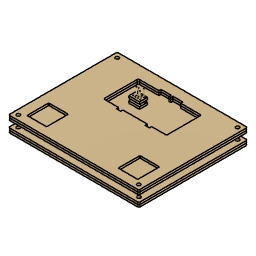
Solum Newton M3 4.3 - Fusion360 (Autodesk Fusion 360 design; units mm, degrees)
Autodesk Fusion 360 part; units mm, degrees
sketch "Skizze1" plane through (0, 0, 0) normal (0, 0, 1) x (1, 0, 0)
  line L0 (-29, 42) -> (-29, 12)
  line L1 (29, 12) -> (29, 42)
  line L2 (-10, 43) -> (-10, 45)
  line L3 (10, 43) -> (10, 45)
  line L4 (10, 45) -> (0.8, 45)
  line L5 (-10, 45) -> (-0.8, 45)
  line L6 (-0.8, 45) -> (-0.8, 43)
  line L7 (0.8, 45) -> (0.8, 43)
  line L8 (-15.25, 9) -> (-15.25, 11)
  line L9 (15.25, 11) -> (15.25, 9)
  line L10 (-11.25, 9) -> (-11.25, 11)
  line L11 (11.25, 11) -> (11.25, 9)
  line L12 (15.25, 9) -> (11.25, 9)
  line L13 (-11.25, 9) -> (-15.25, 9)
  line L14 (15.25, 11) -> (28, 11)
  line L15 (-28, 11) -> (-15.25, 11)
  line L16 (-11.25, 11) -> (11.25, 11)
  arc A0 (-28, 43) -> (-29, 42) centre (-28, 42) ccw
  arc A1 (29, 42) -> (28, 43) centre (28, 42) ccw
  arc A2 (28, 11) -> (29, 12) centre (28, 12) ccw
  arc A3 (-29, 12) -> (-28, 11) centre (-28, 12) ccw
  line L17 (-50.5, -17.5) -> (-33.5, -17.5)
  line L18 (-33, -18) -> (-33, -37)
  line L19 (-33.5, -37.5) -> (-50.5, -37.5)
  line L20 (-51, -37) -> (-51, -18)
  line L21 (51.5, 46) -> (-51.5, 46) construction
  line L22 (-51.5, 46) -> (-51.5, -37) construction
  line L23 (-51.5, -37) -> (51.5, -37) construction
  line L24 (51.5, -37) -> (51.5, 46) construction
  line L25 (51.5, 46) -> (-51.5, -37) construction
  line L26 (-51.5, 46) -> (51.5, -37) construction
  line L27 (50.5, -37.5) -> (33.5, -37.5)
  line L28 (33, -37) -> (33, -18)
  line L29 (33.5, -17.5) -> (50.5, -17.5)
  line L30 (51, -18) -> (51, -37)
  line L31 (-14.05, 36.45) -> (-14.05, 29.15)
  circle A4 centre (-15.75, 35) radius 0.75
  circle A5 centre (-19.95, 35) radius 0.75
  circle A6 centre (-19.95, 31.4) radius 0.75
  circle A7 centre (-16.75, 33.2) radius 0.75
  circle A8 centre (-15.75, 31.4) radius 0.75
  line L32 (-23.85, 36.45) -> (-14.05, 36.45)
  circle A9 centre (-17.85, 31.4) radius 0.75
  circle A10 centre (-17.85, 35) radius 0.75
  line L33 (-23.85, 29.15) -> (-14.05, 36.45) construction
  circle A11 centre (-20.95, 33.2) radius 0.75
  circle A12 centre (-18.85, 33.2) radius 0.75
  circle A13 centre (-22.05, 35) radius 0.75
  circle A14 centre (-22.05, 31.4) radius 0.75
  line L34 (-14.05, 29.15) -> (-23.85, 36.45) construction
  line L35 (-23.85, 29.15) -> (-23.85, 36.45)
  line L36 (-14.05, 29.15) -> (-23.85, 29.15)
  line L37 (59, -45.5) -> (-59, -45.5)
  line L38 (-60, -44.5) -> (-60, 53.5)
  line L39 (-59, 54.5) -> (59, 54.5)
  line L40 (60, 53.5) -> (60, -44.5)
  line L41 (60, -45.5) -> (-60, 54.5) construction
  line L42 (-60, -45.5) -> (60, 54.5) construction
  circle A15 centre (-55.5, 50) radius 1.6
  circle A16 centre (55.5, 50) radius 1.6
  circle A17 centre (-55.5, -41) radius 1.6
  circle A18 centre (55.5, -41) radius 1.6
  line L43 (-10, 43) -> (-28, 43)
  line L44 (28, 43) -> (10, 43)
  line L45 (0.8, 43) -> (-0.8, 43)
  arc A19 (-59, 54.5) -> (-60, 53.5) centre (-59, 53.5) ccw
  arc A20 (60, 53.5) -> (59, 54.5) centre (59, 53.5) ccw
  arc A21 (-60, -44.5) -> (-59, -45.5) centre (-59, -44.5) ccw
  arc A22 (59, -45.5) -> (60, -44.5) centre (59, -44.5) ccw
  arc A23 (-50.5, -17.5) -> (-51, -18) centre (-50.5, -18) ccw
  arc A24 (-33, -18) -> (-33.5, -17.5) centre (-33.5, -18) ccw
  arc A25 (-51, -37) -> (-50.5, -37.5) centre (-50.5, -37) ccw
  arc A26 (-33.5, -37.5) -> (-33, -37) centre (-33.5, -37) ccw
  arc A27 (33.5, -17.5) -> (33, -18) centre (33.5, -18) ccw
  arc A28 (33, -37) -> (33.5, -37.5) centre (33.5, -37) ccw
  arc A29 (51, -18) -> (50.5, -17.5) centre (50.5, -18) ccw
  arc A30 (50.5, -37.5) -> (51, -37) centre (50.5, -37) ccw
  circle A31 centre (-22.05, 35) radius 0.45
  circle A32 centre (-19.95, 35) radius 0.45
  circle A33 centre (-17.85, 35) radius 0.45
  circle A34 centre (-15.75, 35) radius 0.45
  circle A35 centre (-20.95, 33.2) radius 0.45
  circle A36 centre (-18.85, 33.2) radius 0.45
  circle A37 centre (-16.75, 33.2) radius 0.45
  circle A38 centre (-22.05, 31.4) radius 0.45
  circle A39 centre (-19.95, 31.4) radius 0.45
  circle A40 centre (-17.85, 31.4) radius 0.45
  circle A41 centre (-15.75, 31.4) radius 0.45
  line L46 (-14.05, 36.45) -> (-14.05, 43)
  line L47 (-23.85, 36.45) -> (-23.85, 43)
  point P0 (0, 27)
  point P1 (0, 11)
  point P2 (-51, -17.5)
  point P3 (-33, -17.5)
  point P4 (-51, -37.5)
  point P5 (0, 4.5)
  point P6 (51, -17.5)
  point P7 (33, -37.5)
  point P8 (33, -17.5)
  point P9 (-18.95, 32.8)
  point P10 (-18.95, 32.8)
  point P11 (0, 4.5)
  dimension "d6" = 2
  dimension "d7" = 9.2
  dimension "d8" = 9.2
  dimension "d22" = 1
  dimension "d23" = 1
  dimension "d24" = 1
  dimension "d25" = 1
  dimension "d43" = 18
  dimension "d44" = 20
  dimension "d45" = 103
  dimension "d46" = 83
  dimension "d47" = 18
  dimension "d48" = 20
  dimension "d54" = 9.8
  dimension "d55" = 7.3
  dimension "d56" = 1.5
  dimension "d57" = 120
  dimension "d58" = 100
  dimension "d59" = 3.2
  dimension "d60" = 3.2
  dimension "d61" = 3.2
  dimension "d62" = 3.2
  dimension "d69" = 1
  dimension "d70" = 1
  dimension "d71" = 1
  dimension "d72" = 1
  dimension "d73" = 0.5
  dimension "d74" = 0.5
  dimension "d75" = 0.5
  dimension "d76" = 0.5
  dimension "d77" = 0.5
  dimension "d78" = 0.5
  dimension "d79" = 0.5
  dimension "d80" = 0.5
  dimension "d89" = 0.9
  constraint horizontal L44
  constraint perpendicular L0 L44
  constraint parallel L15 L44
  constraint parallel L0 L1
  constraint coincident L2.start L44
  constraint perpendicular L2 L44
  constraint perpendicular L3 L44
  constraint perpendicular L3 L4
  constraint perpendicular L2 L5
  constraint perpendicular L5 L6
  constraint perpendicular L4 L7
  constraint horizontal L12
  constraint perpendicular L8 L12
  constraint coincident L9.start L15
  constraint collinear L12 L13
  constraint collinear L14 L15
  constraint coincident P1 L15
  constraint collinear L15 L16
  constraint tangent A0 L44
  constraint tangent L0 A0
  constraint tangent A1 L44
  constraint tangent L1 A1
  constraint tangent L14 A2
  constraint tangent L1 A2
  constraint tangent L0 A3
  constraint tangent L15 A3
  constraint horizontal L17
  constraint vertical L18
  constraint horizontal L19
  constraint vertical L20
  constraint horizontal L21
  constraint perpendicular L21 L22
  constraint parallel L21 L23
  constraint parallel L22 L24
  constraint coincident L25 P11
  constraint coincident L26 P11
  constraint horizontal L29
  constraint vertical L30
  constraint horizontal L27
  constraint vertical L28
  constraint horizontal L36
  constraint perpendicular L35 L36
  constraint parallel L32 L36
  constraint parallel L31 L35
  constraint coincident P10 L34
  constraint coincident P10 L33
  constraint coincident P10 P9
  constraint equal A5 A13
  constraint equal A10 A13
  constraint equal A4 A13
  constraint equal A12 A13
  constraint equal A7 A13
  constraint equal A13 A14
  constraint equal A9 A13
  constraint equal A8 A13
  constraint horizontal L37
  constraint perpendicular L37 L38
  constraint parallel L37 L39
  constraint parallel L38 L40
  constraint coincident L41 P11
  constraint coincident L42 P11
  constraint coincident P11 P5
  constraint collinear L43 L44
  constraint collinear L44 L45
  constraint coincident L41.end L39
  constraint coincident L41.end L38
  constraint tangent L39 A19
  constraint tangent L38 A19
  constraint coincident L42.end L39
  constraint coincident L42.end L40
  constraint tangent L39 A20
  constraint tangent L40 A20
  constraint coincident L42.start L38
  constraint coincident L42.start L37
  constraint tangent L38 A21
  constraint tangent L37 A21
  constraint coincident L41.start L37
  constraint coincident L41.start L40
  constraint tangent L37 A22
  constraint tangent L40 A22
  constraint coincident P2 L17
  constraint coincident P2 L20
  constraint tangent L17 A23
  constraint tangent L20 A23
  constraint coincident P3 L17
  constraint coincident P3 L18
  constraint tangent L17 A24
  constraint tangent L18 A24
  constraint coincident P4 L20
  constraint coincident P4 L19
  constraint tangent L20 A25
  constraint tangent L19 A25
  constraint tangent L19 A26
  constraint tangent L18 A26
  constraint coincident P8 L28
  constraint coincident P8 L29
  constraint tangent L28 A27
  constraint tangent L29 A27
  constraint coincident P7 L28
  constraint coincident P7 L27
  constraint tangent L28 A28
  constraint tangent L27 A28
  constraint coincident P6 L29
  constraint coincident P6 L30
  constraint tangent L29 A29
  constraint tangent L30 A29
  constraint tangent L27 A30
  constraint tangent L30 A30
  constraint concentric A13 A31
  constraint concentric A5 A32
  constraint concentric A10 A33
  constraint concentric A4 A34
  constraint concentric A11 A35
  constraint concentric A12 A36
  constraint concentric A7 A37
  constraint concentric A14 A38
  constraint concentric A6 A39
  constraint concentric A9 A40
  constraint concentric A8 A41
  constraint equal A31 A32
  constraint equal A31 A33
  constraint equal A31 A34
  constraint equal A31 A35
  constraint equal A31 A36
  constraint equal A31 A37
  constraint equal A31 A38
  constraint equal A31 A39
  constraint equal A31 A40
  constraint equal A31 A41
  constraint coincident L43 L46.end
  constraint perpendicular L43 L46
  constraint coincident L43 L47.end
  constraint perpendicular L43 L47
  measures "d6" distance of L2.start L2.end
  measures "d7" distance of L3.end L4.end
  measures "d8" distance of L2.end L5.end
  measures "d22" radius of A0
  measures "d23" radius of A1
  measures "d24" radius of A2
  measures "d25" radius of A3
  measures "d43" distance of P2 P3
  measures "d44" distance of P2 P4
  measures "d45" distance of L22.end L23.end
  measures "d46" distance of L21.end L22.end
  measures "d47" distance of P6 P8
  measures "d48" distance of P7 P8
  measures "d54" distance of L31.start L32.start
  measures "d55" distance of L33.start L32.start
  measures "d56" diameter of A13
  measures "d57" distance of L41.end L42.end
  measures "d58" distance of L42.start L41.end
  measures "d59" diameter of A15
  measures "d60" diameter of A16
  measures "d61" diameter of A17
  measures "d62" diameter of A18
  measures "d69" radius of A19
  measures "d70" radius of A20
  measures "d71" radius of A21
  measures "d72" radius of A22
  measures "d73" radius of A23
  measures "d74" radius of A24
  measures "d75" radius of A25
  measures "d76" radius of A26
  measures "d77" radius of A27
  measures "d78" radius of A28
  measures "d79" radius of A29
  measures "d80" radius of A30
  measures "d89" diameter of A31
extrude "Extrusion20" add sketch "Skizze1" along normal blind 2 contours L0 L1 L2 L3 L4 L5 L6 L7 L8 L9 L10 L11 L12 L13 L14 L15 L16 A0 A1 A2 A3 L31 L35 L36 L43 L44 L45 L46 L47 | L32 L43 L46 L47 | L31 L32 L35 L36 | L17 L18 L19 L20 A23 A24 A25 A26 | L27 L28 L29 L30 A27 A28 A29 A30 | A4 | A5 | A6 | A7 | A8 | A9 | A10 | A11 | A12 | A13 | A14 | L37 L38 L39 L40 A19 A20 A21 A22 | A31 | A32 | A33 | A34 | A35 | A36 | A37 | A38 | A39 | A40 | A41 makes body 1
extrude "Extrusion21" add sketch "Skizze1" along normal blind 2 separate body contours L0 L1 L2 L3 L4 L5 L6 L7 L8 L9 L10 L11 L12 L13 L14 L15 L16 A0 A1 A2 A3 L31 L35 L36 L43 L44 L45 L46 L47 | L32 L43 L46 L47 | L31 L32 L35 L36 | L17 L18 L19 L20 A23 A24 A25 A26 | L27 L28 L29 L30 A27 A28 A29 A30 | A4 | A5 | A6 | A7 | A8 | A9 | A10 | A11 | A12 | A13 | A14 | L37 L38 L39 L40 A19 A20 A21 A22 makes body 2
move_body "Verschieben10" bodies 2 to x (1, 0, 0) y (0, 1, 0) z (0, 0, 1) at (0, 0, 2)
extrude "Extrusion25" add sketch "Skizze1" along normal blind 2 separate body contours L31 L32 L35 L36 | A4 | A5 | A6 | A7 | A8 | A9 | A10 | A11 | A12 | A13 | A14 makes body 3
move_body "Verschieben15" bodies 3 to x (1, 0, 0) y (0, 1, 0) z (0, 0, 1) at (0, 0, 4)
copy_body "Körper kopieren/einfügen4" bodies 3 makes body 4
move_body "Verschieben16" bodies 4 to x (1, 0, 0) y (0, 1, 0) z (0, 0, 1) at (0, 0, 4)
extrude "Extrusion26" add sketch "Skizze1" along normal blind 2 separate body contours L17 L18 L19 L20 A23 A24 A25 A26 | L27 L28 L29 L30 A27 A28 A29 A30 | L37 L38 L39 L40 A19 A20 A21 A22 makes body 5
move_body "Verschieben17" bodies 5 to x (1, 0, 0) y (0, 1, 0) z (0, 0, 1) at (0, 0, 10)
extrude "Extrusion27" add sketch "Skizze1" along normal blind 2 separate body contours L37 L38 L39 L40 A19 A20 A21 A22 makes body 6
move_body "Verschieben18" bodies 6 to x (1, 0, 0) y (0, 1, 0) z (0, 0, 1) at (0, 0, 12)
extrude "Extrusion28" add sketch "Skizze1" along normal blind 15 separate body contours A34 | A35 | A36 | A41 makes body 7 at (-16.1087, 31.6717, 10) makes body 8 at (-19.2978, 33.1552, 10) makes body 9 at (-15.3353, 35.1748, 10) makes body 10 at (-21.3978, 33.1552, 10)
move_body "Verschieben19" bodies 7 8 10 9 to x (1, 0, 0) y (0, 1, 0) z (0, 0, 1) at (0, 0, 2)
chamfer "Fase1" distance 0.3 angle 45 4 faces at (-15.5165, 34.9155, 17) (-18.8834, 33.3462, 17) (-15.8444, 31.6586, 17) (-20.9834, 33.3462, 17) on bodies 7 8 9 10
sketch "Skizze21" plane through (0, 0, 4) normal (0, 0, 1) x (-1, 0, 0)
  circle A0 centre (17.85, -31.4) radius 0.45
  circle A1 centre (18.85, -33.2) radius 0.45
  circle A2 centre (-55.5, -50) radius 1.6
  circle A3 centre (55.5, 41) radius 1.6
  circle A4 centre (22.05, -35) radius 0.45
  circle A5 centre (20.95, -33.2) radius 0.45
  circle A6 centre (19.95, -35) radius 0.45
  circle A7 centre (22.05, -31.4) radius 0.45
  circle A8 centre (15.75, -35) radius 0.45
  circle A9 centre (17.85, -35) radius 0.45
  circle A10 centre (15.75, -31.4) radius 0.45
  circle A11 centre (16.75, -33.2) radius 0.45
  circle A12 centre (55.5, -50) radius 1.6
  circle A13 centre (-55.5, 41) radius 1.6
  circle A14 centre (19.95, -31.4) radius 0.45
  arc A15 (60, 44.5) -> (59, 45.5) centre (59, 44.5) ccw
  line L0 (59, 45.5) -> (-59, 45.5)
  arc A16 (-59, 45.5) -> (-60, 44.5) centre (-59, 44.5) ccw
  line L1 (-60, 44.5) -> (-60, -53.5)
  arc A17 (-60, -53.5) -> (-59, -54.5) centre (-59, -53.5) ccw
  line L2 (-59, -54.5) -> (59, -54.5)
  arc A18 (59, -54.5) -> (60, -53.5) centre (59, -53.5) ccw
  line L3 (60, -53.5) -> (60, 44.5)
sketch "Skizze20" plane through (0, 0, 14) normal (0, 0, 1) x (-1, 0, 0)
  circle A0 centre (55.5, -50) radius 1.6
  line L0 (-28, -11) -> (-15.25, -11)
  line L1 (-15.25, -11) -> (-15.25, -9)
  line L2 (-15.25, -9) -> (-11.25, -9)
  line L3 (-11.25, -9) -> (-11.25, -11)
  line L4 (-11.25, -11) -> (11.25, -11)
  line L5 (11.25, -11) -> (11.25, -9)
  line L6 (11.25, -9) -> (15.25, -9)
  line L7 (15.25, -9) -> (15.25, -11)
  line L8 (15.25, -11) -> (28, -11)
  arc A1 (29, -12) -> (28, -11) centre (28, -12) ccw
  line L9 (29, -12) -> (29, -42)
  arc A2 (28, -43) -> (29, -42) centre (28, -42) ccw
  line L10 (28, -43) -> (10, -43)
  line L11 (10, -43) -> (10, -45)
  line L12 (10, -45) -> (0.8, -45)
  line L13 (0.8, -45) -> (0.8, -43)
  line L14 (0.8, -43) -> (-0.8, -43)
  line L15 (-0.8, -43) -> (-0.8, -45)
  line L16 (-0.8, -45) -> (-10, -45)
  line L17 (-10, -45) -> (-10, -43)
  line L18 (-10, -43) -> (-28, -43)
  arc A3 (-29, -42) -> (-28, -43) centre (-28, -42) ccw
  line L19 (-29, -42) -> (-29, -12)
  arc A4 (-28, -11) -> (-29, -12) centre (-28, -12) ccw
  circle A5 centre (-55.5, -50) radius 1.6
  arc A6 (51, 37) -> (50.5, 37.5) centre (50.5, 37) ccw
  line L20 (51, 37) -> (51, 18)
  arc A7 (50.5, 17.5) -> (51, 18) centre (50.5, 18) ccw
  line L21 (50.5, 17.5) -> (33.5, 17.5)
  arc A8 (33, 18) -> (33.5, 17.5) centre (33.5, 18) ccw
  line L22 (33, 18) -> (33, 37)
  arc A9 (33.5, 37.5) -> (33, 37) centre (33.5, 37) ccw
  line L23 (33.5, 37.5) -> (50.5, 37.5)
  circle A10 centre (55.5, 41) radius 1.6
  circle A11 centre (-55.5, 41) radius 1.6
  arc A12 (-33, 37) -> (-33.5, 37.5) centre (-33.5, 37) ccw
  line L24 (-33, 37) -> (-33, 18)
  arc A13 (-33.5, 17.5) -> (-33, 18) centre (-33.5, 18) ccw
  line L25 (-33.5, 17.5) -> (-50.5, 17.5)
  arc A14 (-51, 18) -> (-50.5, 17.5) centre (-50.5, 18) ccw
  line L26 (-51, 18) -> (-51, 37)
  arc A15 (-50.5, 37.5) -> (-51, 37) centre (-50.5, 37) ccw
  line L27 (-50.5, 37.5) -> (-33.5, 37.5)
  arc A16 (60, 44.5) -> (59, 45.5) centre (59, 44.5) ccw
  line L28 (59, 45.5) -> (-59, 45.5)
  arc A17 (-59, 45.5) -> (-60, 44.5) centre (-59, 44.5) ccw
  line L29 (-60, 44.5) -> (-60, -53.5)
  arc A18 (-60, -53.5) -> (-59, -54.5) centre (-59, -53.5) ccw
  line L30 (-59, -54.5) -> (59, -54.5)
  arc A19 (59, -54.5) -> (60, -53.5) centre (59, -53.5) ccw
  line L31 (60, -53.5) -> (60, 44.5)
sketch "Skizze19" plane through (0, 0, 12) normal (0, 0, 1) x (-1, 0, 0)
  line L0 (-28, -11) -> (-15.25, -11)
  line L1 (-15.25, -11) -> (-15.25, -9)
  line L2 (-15.25, -9) -> (-11.25, -9)
  line L3 (-11.25, -9) -> (-11.25, -11)
  line L4 (-11.25, -11) -> (11.25, -11)
  line L5 (11.25, -11) -> (11.25, -9)
  line L6 (11.25, -9) -> (15.25, -9)
  line L7 (15.25, -9) -> (15.25, -11)
  line L8 (15.25, -11) -> (28, -11)
  arc A0 (29, -12) -> (28, -11) centre (28, -12) ccw
  line L9 (29, -12) -> (29, -42)
  arc A1 (28, -43) -> (29, -42) centre (28, -42) ccw
  line L10 (28, -43) -> (10, -43)
  line L11 (10, -43) -> (10, -45)
  line L12 (10, -45) -> (0.8, -45)
  line L13 (0.8, -45) -> (0.8, -43)
  line L14 (0.8, -43) -> (-0.8, -43)
  line L15 (-0.8, -43) -> (-0.8, -45)
  line L16 (-0.8, -45) -> (-10, -45)
  line L17 (-10, -45) -> (-10, -43)
  line L18 (-10, -43) -> (-28, -43)
  arc A2 (-29, -42) -> (-28, -43) centre (-28, -42) ccw
  line L19 (-29, -42) -> (-29, -12)
  arc A3 (-28, -11) -> (-29, -12) centre (-28, -12) ccw
  circle A4 centre (-55.5, -50) radius 1.6
  circle A5 centre (55.5, -50) radius 1.6
  circle A6 centre (55.5, 41) radius 1.6
  circle A7 centre (-55.5, 41) radius 1.6
  arc A8 (60, 44.5) -> (59, 45.5) centre (59, 44.5) ccw
  line L20 (59, 45.5) -> (-59, 45.5)
  arc A9 (-59, 45.5) -> (-60, 44.5) centre (-59, 44.5) ccw
  line L21 (-60, 44.5) -> (-60, -53.5)
  arc A10 (-60, -53.5) -> (-59, -54.5) centre (-59, -53.5) ccw
  line L22 (-59, -54.5) -> (59, -54.5)
  arc A11 (59, -54.5) -> (60, -53.5) centre (59, -53.5) ccw
  line L23 (60, -53.5) -> (60, 44.5)
sketch "Skizze18" plane through (0, 0, 8) normal (0, 0, 1) x (-1, 0, 0)
  circle A0 centre (20.95, -35) radius 0.45
  circle A1 centre (18.85, -35) radius 0.45
  circle A2 centre (16.75, -31.4) radius 0.45
  circle A3 centre (23.05, -35) radius 0.45
  circle A4 centre (16.75, -35) radius 0.45
  circle A5 centre (18.85, -31.4) radius 0.45
  circle A6 centre (20.95, -31.4) radius 0.45
  circle A7 centre (19.85, -33.2) radius 0.45
  circle A8 centre (21.95, -33.2) radius 0.45
  circle A9 centre (17.75, -33.2) radius 0.45
  circle A10 centre (23.05, -31.4) radius 0.45
  line L0 (15.05, -29.15) -> (15.05, -36.45)
  line L1 (15.05, -36.45) -> (24.85, -36.45)
  line L2 (24.85, -36.45) -> (24.85, -29.15)
  line L3 (24.85, -29.15) -> (15.05, -29.15)
sketch "Skizze17" plane through (0, 0, 4) normal (0, 0, 1) x (-1, 0, 0)
  circle A0 centre (23.05, -31.4) radius 0.45
  circle A1 centre (23.05, -35) radius 0.45
  circle A2 centre (18.85, -35) radius 0.45
  circle A3 centre (-55.5, -50) radius 1.6
  circle A4 centre (55.5, 41) radius 1.6
  circle A5 centre (16.75, -31.4) radius 0.45
  circle A6 centre (16.75, -35) radius 0.45
  circle A7 centre (17.75, -33.2) radius 0.45
  circle A8 centre (20.95, -31.4) radius 0.45
  circle A9 centre (55.5, -50) radius 1.6
  circle A10 centre (19.85, -33.2) radius 0.45
  circle A11 centre (21.95, -33.2) radius 0.45
  circle A12 centre (18.85, -31.4) radius 0.45
  circle A13 centre (-55.5, 41) radius 1.6
  circle A14 centre (20.95, -35) radius 0.45
  arc A15 (60, 44.5) -> (59, 45.5) centre (59, 44.5) ccw
  line L0 (59, 45.5) -> (-59, 45.5)
  arc A16 (-59, 45.5) -> (-60, 44.5) centre (-59, 44.5) ccw
  line L1 (-60, 44.5) -> (-60, -53.5)
  arc A17 (-60, -53.5) -> (-59, -54.5) centre (-59, -53.5) ccw
  line L2 (-59, -54.5) -> (59, -54.5)
  arc A18 (59, -54.5) -> (60, -53.5) centre (59, -53.5) ccw
  line L3 (60, -53.5) -> (60, 44.5)
sketch "Skizze16" plane through (0, 0, 2) normal (0, 0, 1) x (-1, 0, 0)
  circle A0 centre (-55.5, -50) radius 1.6
  circle A1 centre (-55.5, 41) radius 1.6
  circle A2 centre (55.5, 41) radius 1.6
  circle A3 centre (55.5, -50) radius 1.6
  arc A4 (60, 44.5) -> (59, 45.5) centre (59, 44.5) ccw
  line L0 (59, 45.5) -> (-59, 45.5)
  arc A5 (-59, 45.5) -> (-60, 44.5) centre (-59, 44.5) ccw
  line L1 (-60, 44.5) -> (-60, -53.5)
  arc A6 (-60, -53.5) -> (-59, -54.5) centre (-59, -53.5) ccw
  line L2 (-59, -54.5) -> (59, -54.5)
  arc A7 (59, -54.5) -> (60, -53.5) centre (59, -53.5) ccw
  line L3 (60, -53.5) -> (60, 44.5)
extrude "Extrusion22" [suppressed]
move_body "Verschieben11" [suppressed]
extrude "Extrusion23" [suppressed]
move_body "Verschieben12" [suppressed]
extrude "Extrusion24" [suppressed]
move_body "Verschieben13" [suppressed]
copy_body "Körper kopieren/einfügen3" [suppressed]
move_body "Verschieben14" [suppressed]
extrude "Extrusion15" [suppressed]
copy_body "Körper kopieren/einfügen1" [suppressed]
move_body "Verschieben1" [suppressed]
extrude "Extrusion16" [suppressed]
move_body "Verschieben2" [suppressed]
move_body "Verschieben3" [suppressed]
extrude "Extrusion17" [suppressed]
move_body "Verschieben4" [suppressed]
copy_body "Körper kopieren/einfügen2" [suppressed]
move_body "Verschieben5" [suppressed]
extrude "Extrusion18" [suppressed]
move_body "Verschieben6" [suppressed]
move_body "Verschieben7" [suppressed]
extrude "Extrusion19" [suppressed]
delete_body "Körper entfernen1" bodies 11
move_body "Verschieben8" [suppressed]
move_body "Verschieben9" [suppressed]
extrude "Extrusion14" [suppressed]
extrude "Extrusion13" [suppressed]
sketch "Skizze15" plane through (0, 0, 2) normal (0, 0, 1) x (-1, 0, 0)
  circle A0 centre (-55.5, -50) radius 1.6
  circle A1 centre (-18.3, -33.2) radius 0.45
  circle A2 centre (-55.5, 41) radius 1.6
  circle A3 centre (-23.5, -31.4) radius 0.45
  circle A4 centre (55.5, -50) radius 1.6
  circle A5 centre (-17.2, -35) radius 0.45
  circle A6 centre (-21.4, -31.4) radius 0.45
  circle A7 centre (-19.3, -31.4) radius 0.45
  circle A8 centre (-21.4, -35) radius 0.45
  circle A9 centre (-22.5, -33.2) radius 0.45
  circle A10 centre (-17.2, -31.4) radius 0.45
  circle A11 centre (-19.3, -35) radius 0.45
  circle A12 centre (55.5, 41) radius 1.6
  circle A13 centre (-20.4, -33.2) radius 0.45
  circle A14 centre (-23.5, -35) radius 0.45
  arc A15 (60, 44.5) -> (59, 45.5) centre (59, 44.5) ccw
  line L0 (59, 45.5) -> (-59, 45.5)
  arc A16 (-59, 45.5) -> (-60, 44.5) centre (-59, 44.5) ccw
  line L1 (-60, 44.5) -> (-60, -53.5)
  arc A17 (-60, -53.5) -> (-59, -54.5) centre (-59, -53.5) ccw
  line L2 (-59, -54.5) -> (59, -54.5)
  arc A18 (59, -54.5) -> (60, -53.5) centre (59, -53.5) ccw
  line L3 (60, -53.5) -> (60, 44.5)
extrude "Extrusion12" [suppressed]
sketch "Skizze14" plane through (0, 0, 2) normal (0, 0, 1) x (-1, 0, 0)
  circle A0 centre (55.5, -50) radius 1.6
  circle A1 centre (-55.5, 41) radius 1.6
  circle A2 centre (55.5, 41) radius 1.6
  line L0 (-28, -11) -> (-15.25, -11)
  line L1 (-15.25, -11) -> (-15.25, -9)
  line L2 (-15.25, -9) -> (-11.25, -9)
  line L3 (-11.25, -9) -> (-11.25, -11)
  line L4 (-11.25, -11) -> (11.25, -11)
  line L5 (11.25, -11) -> (11.25, -9)
  line L6 (11.25, -9) -> (15.25, -9)
  line L7 (15.25, -9) -> (15.25, -11)
  line L8 (15.25, -11) -> (28, -11)
  arc A3 (29, -12) -> (28, -11) centre (28, -12) ccw
  line L9 (29, -12) -> (29, -42)
  arc A4 (28, -43) -> (29, -42) centre (28, -42) ccw
  line L10 (28, -43) -> (10, -43)
  line L11 (10, -43) -> (10, -45)
  line L12 (10, -45) -> (0.8, -45)
  line L13 (0.8, -45) -> (0.8, -43)
  line L14 (0.8, -43) -> (-0.8, -43)
  line L15 (-0.8, -43) -> (-0.8, -45)
  line L16 (-0.8, -45) -> (-10, -45)
  line L17 (-10, -45) -> (-10, -43)
  line L18 (-10, -43) -> (-28, -43)
  arc A5 (-29, -42) -> (-28, -43) centre (-28, -42) ccw
  line L19 (-29, -42) -> (-29, -12)
  arc A6 (-28, -11) -> (-29, -12) centre (-28, -12) ccw
  circle A7 centre (-55.5, -50) radius 1.6
  arc A8 (60, 44.5) -> (59, 45.5) centre (59, 44.5) ccw
  line L20 (59, 45.5) -> (-59, 45.5)
  arc A9 (-59, 45.5) -> (-60, 44.5) centre (-59, 44.5) ccw
  line L21 (-60, 44.5) -> (-60, -53.5)
  arc A10 (-60, -53.5) -> (-59, -54.5) centre (-59, -53.5) ccw
  line L22 (-59, -54.5) -> (59, -54.5)
  arc A11 (59, -54.5) -> (60, -53.5) centre (59, -53.5) ccw
  line L23 (60, -53.5) -> (60, 44.5)
extrude "Extrusion11" [suppressed]
sketch "Skizze13" plane through (0, 0, 2) normal (0, 0, 1) x (-1, 0, 0)
  circle A0 centre (55.5, -50) radius 1.6
  arc A1 (-33, 37) -> (-33.5, 37.5) centre (-33.5, 37) ccw
  line L0 (-33, 37) -> (-33, 18)
  arc A2 (-33.5, 17.5) -> (-33, 18) centre (-33.5, 18) ccw
  line L1 (-33.5, 17.5) -> (-50.5, 17.5)
  arc A3 (-51, 18) -> (-50.5, 17.5) centre (-50.5, 18) ccw
  line L2 (-51, 18) -> (-51, 37)
  arc A4 (-50.5, 37.5) -> (-51, 37) centre (-50.5, 37) ccw
  line L3 (-50.5, 37.5) -> (-33.5, 37.5)
  circle A5 centre (-55.5, 41) radius 1.6
  arc A6 (51, 37) -> (50.5, 37.5) centre (50.5, 37) ccw
  line L4 (51, 37) -> (51, 18)
  arc A7 (50.5, 17.5) -> (51, 18) centre (50.5, 18) ccw
  line L5 (50.5, 17.5) -> (33.5, 17.5)
  arc A8 (33, 18) -> (33.5, 17.5) centre (33.5, 18) ccw
  line L6 (33, 18) -> (33, 37)
  arc A9 (33.5, 37.5) -> (33, 37) centre (33.5, 37) ccw
  line L7 (33.5, 37.5) -> (50.5, 37.5)
  line L8 (-28, -11) -> (-15.25, -11)
  line L9 (-15.25, -11) -> (-15.25, -9)
  line L10 (-15.25, -9) -> (-11.25, -9)
  line L11 (-11.25, -9) -> (-11.25, -11)
  line L12 (-11.25, -11) -> (11.25, -11)
  line L13 (11.25, -11) -> (11.25, -9)
  line L14 (11.25, -9) -> (15.25, -9)
  line L15 (15.25, -9) -> (15.25, -11)
  line L16 (15.25, -11) -> (28, -11)
  arc A10 (29, -12) -> (28, -11) centre (28, -12) ccw
  line L17 (29, -12) -> (29, -42)
  arc A11 (28, -43) -> (29, -42) centre (28, -42) ccw
  line L18 (28, -43) -> (10, -43)
  line L19 (10, -43) -> (10, -45)
  line L20 (10, -45) -> (0.8, -45)
  line L21 (0.8, -45) -> (0.8, -43)
  line L22 (0.8, -43) -> (-0.8, -43)
  line L23 (-0.8, -43) -> (-0.8, -45)
  line L24 (-0.8, -45) -> (-10, -45)
  line L25 (-10, -45) -> (-10, -43)
  line L26 (-10, -43) -> (-28, -43)
  arc A12 (-29, -42) -> (-28, -43) centre (-28, -42) ccw
  line L27 (-29, -42) -> (-29, -12)
  arc A13 (-28, -11) -> (-29, -12) centre (-28, -12) ccw
  circle A14 centre (55.5, 41) radius 1.6
  circle A15 centre (-55.5, -50) radius 1.6
  arc A16 (60, 44.5) -> (59, 45.5) centre (59, 44.5) ccw
  line L28 (59, 45.5) -> (-59, 45.5)
  arc A17 (-59, 45.5) -> (-60, 44.5) centre (-59, 44.5) ccw
  line L29 (-60, 44.5) -> (-60, -53.5)
  arc A18 (-60, -53.5) -> (-59, -54.5) centre (-59, -53.5) ccw
  line L30 (-59, -54.5) -> (59, -54.5)
  arc A19 (59, -54.5) -> (60, -53.5) centre (59, -53.5) ccw
  line L31 (60, -53.5) -> (60, 44.5)
extrude "Extrusion10" [suppressed]
sketch "Skizze12" plane through (0, 0, 2) normal (0, 0, 1) x (-1, 0, 0)
  circle A0 centre (55.5, 41) radius 1.6
  circle A1 centre (-23.5, -35) radius 0.75
  circle A2 centre (-19.3, -35) radius 0.75
  circle A3 centre (-20.4, -33.2) radius 0.75
  circle A4 centre (-23.5, -31.4) radius 0.75
  circle A5 centre (-22.5, -33.2) radius 0.75
  circle A6 centre (-21.4, -35) radius 0.75
  circle A7 centre (-19.3, -31.4) radius 0.75
  circle A8 centre (55.5, -50) radius 1.6
  circle A9 centre (-18.3, -33.2) radius 0.75
  circle A10 centre (-17.2, -35) radius 0.75
  circle A11 centre (-17.2, -31.4) radius 0.75
  circle A12 centre (-55.5, -50) radius 1.6
  circle A13 centre (-21.4, -31.4) radius 0.75
  circle A14 centre (-55.5, 41) radius 1.6
  arc A15 (60, 44.5) -> (59, 45.5) centre (59, 44.5) ccw
  line L0 (59, 45.5) -> (-59, 45.5)
  arc A16 (-59, 45.5) -> (-60, 44.5) centre (-59, 44.5) ccw
  line L1 (-60, 44.5) -> (-60, -53.5)
  arc A17 (-60, -53.5) -> (-59, -54.5) centre (-59, -53.5) ccw
  line L2 (-59, -54.5) -> (59, -54.5)
  arc A18 (59, -54.5) -> (60, -53.5) centre (59, -53.5) ccw
  line L3 (60, -53.5) -> (60, 44.5)
extrude "Extrusion9" [suppressed]
sketch "Skizze11" plane through (0, 0, 2) normal (0, 0, 1) x (-1, 0, 0)
  circle A0 centre (-55.5, -50) radius 1.6
  arc A1 (-33, 37) -> (-33.5, 37.5) centre (-33.5, 37) ccw
  line L0 (-33, 37) -> (-33, 18)
  arc A2 (-33.5, 17.5) -> (-33, 18) centre (-33.5, 18) ccw
  line L1 (-33.5, 17.5) -> (-50.5, 17.5)
  arc A3 (-51, 18) -> (-50.5, 17.5) centre (-50.5, 18) ccw
  line L2 (-51, 18) -> (-51, 37)
  arc A4 (-50.5, 37.5) -> (-51, 37) centre (-50.5, 37) ccw
  line L3 (-50.5, 37.5) -> (-33.5, 37.5)
  arc A5 (51, 37) -> (50.5, 37.5) centre (50.5, 37) ccw
  line L4 (51, 37) -> (51, 18)
  arc A6 (50.5, 17.5) -> (51, 18) centre (50.5, 18) ccw
  line L5 (50.5, 17.5) -> (33.5, 17.5)
  arc A7 (33, 18) -> (33.5, 17.5) centre (33.5, 18) ccw
  line L6 (33, 18) -> (33, 37)
  arc A8 (33.5, 37.5) -> (33, 37) centre (33.5, 37) ccw
  line L7 (33.5, 37.5) -> (50.5, 37.5)
  circle A9 centre (55.5, -50) radius 1.6
  circle A10 centre (55.5, 41) radius 1.6
  line L8 (-28, -11) -> (-15.25, -11)
  line L9 (-15.25, -11) -> (-15.25, -9)
  line L10 (-15.25, -9) -> (-11.25, -9)
  line L11 (-11.25, -9) -> (-11.25, -11)
  line L12 (-11.25, -11) -> (11.25, -11)
  line L13 (11.25, -11) -> (11.25, -9)
  line L14 (11.25, -9) -> (15.25, -9)
  line L15 (15.25, -9) -> (15.25, -11)
  line L16 (15.25, -11) -> (28, -11)
  arc A11 (29, -12) -> (28, -11) centre (28, -12) ccw
  line L17 (29, -12) -> (29, -42)
  arc A12 (28, -43) -> (29, -42) centre (28, -42) ccw
  line L18 (28, -43) -> (10, -43)
  line L19 (10, -43) -> (10, -45)
  line L20 (10, -45) -> (0.8, -45)
  line L21 (0.8, -45) -> (0.8, -43)
  line L22 (0.8, -43) -> (-0.8, -43)
  line L23 (-0.8, -43) -> (-0.8, -45)
  line L24 (-0.8, -45) -> (-10, -45)
  line L25 (-10, -45) -> (-10, -43)
  line L26 (-10, -43) -> (-28, -43)
  arc A13 (-29, -42) -> (-28, -43) centre (-28, -42) ccw
  line L27 (-29, -42) -> (-29, -12)
  arc A14 (-28, -11) -> (-29, -12) centre (-28, -12) ccw
  circle A15 centre (-55.5, 41) radius 1.6
  arc A16 (60, 44.5) -> (59, 45.5) centre (59, 44.5) ccw
  line L28 (59, 45.5) -> (-59, 45.5)
  arc A17 (-59, 45.5) -> (-60, 44.5) centre (-59, 44.5) ccw
  line L29 (-60, 44.5) -> (-60, -53.5)
  arc A18 (-60, -53.5) -> (-59, -54.5) centre (-59, -53.5) ccw
  line L30 (-59, -54.5) -> (59, -54.5)
  arc A19 (59, -54.5) -> (60, -53.5) centre (59, -53.5) ccw
  line L31 (60, -53.5) -> (60, 44.5)
extrude "Extrusion8" [suppressed]
sketch "Skizze10" plane through (0, 0, 2) normal (0, 0, 1) x (-1, 0, 0)
  circle A0 centre (-19.3, -35) radius 0.75
  circle A1 centre (-21.4, -31.4) radius 0.75
  circle A2 centre (-55.5, -50) radius 1.6
  circle A3 centre (55.5, -50) radius 1.6
  circle A4 centre (-17.2, -31.4) radius 0.75
  circle A5 centre (-20.4, -33.2) radius 0.75
  circle A6 centre (-17.2, -35) radius 0.75
  circle A7 centre (-18.3, -33.2) radius 0.75
  circle A8 centre (-23.5, -31.4) radius 0.75
  circle A9 centre (-22.5, -33.2) radius 0.75
  circle A10 centre (-21.4, -35) radius 0.75
  circle A11 centre (-55.5, 41) radius 1.6
  circle A12 centre (55.5, 41) radius 1.6
  circle A13 centre (-19.3, -31.4) radius 0.75
  circle A14 centre (-23.5, -35) radius 0.75
  line L0 (-60, -54.5) -> (60, -54.5)
  line L1 (60, -54.5) -> (60, 45.5)
  line L2 (60, 45.5) -> (-60, 45.5)
  line L3 (-60, 45.5) -> (-60, -54.5)
extrude "Extrusion7" [suppressed]
extrude "Extrusion6" [suppressed]
sketch "Skizze9" plane through (0, 0, 2) normal (0, 0, 1) x (-1, 0, 0)
  circle A0 centre (55.5, -50) radius 1.6
  circle A1 centre (-55.5, -50) radius 1.6
  line L0 (-33, 17.5) -> (-51, 17.5)
  line L1 (-51, 17.5) -> (-51, 37.5)
  line L2 (-51, 37.5) -> (-33, 37.5)
  line L3 (-33, 37.5) -> (-33, 17.5)
  line L4 (33, 37.5) -> (51, 37.5)
  line L5 (51, 37.5) -> (51, 17.5)
  line L6 (51, 17.5) -> (33, 17.5)
  line L7 (33, 17.5) -> (33, 37.5)
  circle A2 centre (55.5, 41) radius 1.6
  circle A3 centre (-55.5, 41) radius 1.6
  line L8 (-28, -11) -> (-15.25, -11)
  line L9 (-15.25, -11) -> (-15.25, -9)
  line L10 (-15.25, -9) -> (-11.25, -9)
  line L11 (-11.25, -9) -> (-11.25, -11)
  line L12 (-11.25, -11) -> (11.25, -11)
  line L13 (11.25, -11) -> (11.25, -9)
  line L14 (11.25, -9) -> (15.25, -9)
  line L15 (15.25, -9) -> (15.25, -11)
  line L16 (15.25, -11) -> (28, -11)
  arc A4 (29, -12) -> (28, -11) centre (28, -12) ccw
  line L17 (29, -12) -> (29, -42)
  arc A5 (28, -43) -> (29, -42) centre (28, -42) ccw
  line L18 (28, -43) -> (10, -43)
  line L19 (10, -43) -> (10, -45)
  line L20 (10, -45) -> (0.8, -45)
  line L21 (0.8, -45) -> (0.8, -43)
  line L22 (0.8, -43) -> (-0.8, -43)
  line L23 (-0.8, -43) -> (-0.8, -45)
  line L24 (-0.8, -45) -> (-10, -45)
  line L25 (-10, -45) -> (-10, -43)
  line L26 (-10, -43) -> (-28, -43)
  arc A6 (-29, -42) -> (-28, -43) centre (-28, -42) ccw
  line L27 (-29, -42) -> (-29, -12)
  arc A7 (-28, -11) -> (-29, -12) centre (-28, -12) ccw
  line L28 (-60, -54.5) -> (60, -54.5)
  line L29 (60, -54.5) -> (60, 45.5)
  line L30 (60, 45.5) -> (-60, 45.5)
  line L31 (-60, 45.5) -> (-60, -54.5)
extrude "Extrusion5" [suppressed]
sketch "Skizze8" plane through (0, 0, 2) normal (0, 0, 1) x (-1, 0, 0)
  circle A0 centre (54, -44) radius 1.6
  circle A1 centre (54, 44) radius 1.6
  circle A2 centre (-21.47, -35) radius 0.45
  circle A3 centre (-20.455, -32.97) radius 0.45
  circle A4 centre (-22.485, -32.97) radius 0.45
  circle A5 centre (-17.41, -30.94) radius 0.45
  circle A6 centre (-19.44, -35) radius 0.45
  circle A7 centre (-23.5, -35) radius 0.45
  circle A8 centre (-23.5, -30.94) radius 0.45
  circle A9 centre (-18.425, -32.97) radius 0.45
  circle A10 centre (-54, 44) radius 1.6
  circle A11 centre (-17.41, -35) radius 0.45
  circle A12 centre (-19.44, -30.94) radius 0.45
  circle A13 centre (-21.47, -30.94) radius 0.45
  circle A14 centre (-54, -44) radius 1.6
  line L0 (-60, -50) -> (60, -50)
  line L1 (60, -50) -> (60, 50)
  line L2 (60, 50) -> (-60, 50)
  line L3 (-60, 50) -> (-60, -50)
extrude "Extrusion4" [suppressed]
sketch "Skizze7" plane through (0, 0, 2) normal (0, 0, 1) x (-1, 0, 0)
  circle A0 centre (-54, 44) radius 1.6
  circle A1 centre (-54, -44) radius 1.6
  circle A2 centre (54, 44) radius 1.6
  line L0 (33, 37.5) -> (52, 37.5)
  line L1 (52, 37.5) -> (52, 17.5)
  line L2 (52, 17.5) -> (33, 17.5)
  line L3 (33, 17.5) -> (33, 37.5)
  line L4 (-33, 17.5) -> (-52, 17.5)
  line L5 (-52, 17.5) -> (-52, 37.5)
  line L6 (-52, 37.5) -> (-33, 37.5)
  line L7 (-33, 37.5) -> (-33, 17.5)
  line L8 (28, -43) -> (10, -43)
  line L9 (10, -43) -> (10, -45)
  line L10 (10, -45) -> (0.8, -45)
  line L11 (0.8, -45) -> (0.8, -43)
  line L12 (0.8, -43) -> (-0.8, -43)
  line L13 (-0.8, -43) -> (-0.8, -45)
  line L14 (-0.8, -45) -> (-10, -45)
  line L15 (-10, -45) -> (-10, -43)
  line L16 (-10, -43) -> (-28, -43)
  arc A3 (-29, -42) -> (-28, -43) centre (-28, -42) ccw
  line L17 (-29, -42) -> (-29, -12)
  arc A4 (-28, -11) -> (-29, -12) centre (-28, -12) ccw
  line L18 (-28, -11) -> (-15.25, -11)
  line L19 (-15.25, -11) -> (-15.25, -9)
  line L20 (-15.25, -9) -> (-11.25, -9)
  line L21 (-11.25, -9) -> (-11.25, -11)
  line L22 (-11.25, -11) -> (11.25, -11)
  line L23 (11.25, -11) -> (11.25, -9)
  line L24 (11.25, -9) -> (15.25, -9)
  line L25 (15.25, -9) -> (15.25, -11)
  line L26 (15.25, -11) -> (28, -11)
  arc A5 (29, -12) -> (28, -11) centre (28, -12) ccw
  line L27 (29, -12) -> (29, -42)
  arc A6 (28, -43) -> (29, -42) centre (28, -42) ccw
  circle A7 centre (54, -44) radius 1.6
  line L28 (-60, -50) -> (60, -50)
  line L29 (60, -50) -> (60, 50)
  line L30 (60, 50) -> (-60, 50)
  line L31 (-60, 50) -> (-60, -50)
extrude "Extrusion3" [suppressed]
sketch "Skizze6" plane through (0, 0, 2) normal (0, 0, 1) x (-1, 0, 0)
  circle A0 centre (-21.47, -30.94) radius 0.75
  circle A1 centre (54, -44) radius 1.6
  circle A2 centre (-20.455, -32.97) radius 0.75
  circle A3 centre (-23.5, -35) radius 0.75
  circle A4 centre (-19.44, -30.94) radius 0.75
  circle A5 centre (-17.41, -30.94) radius 0.75
  circle A6 centre (-21.47, -35) radius 0.75
  circle A7 centre (54, 44) radius 1.6
  circle A8 centre (-23.5, -30.94) radius 0.75
  circle A9 centre (-19.44, -35) radius 0.75
  circle A10 centre (-54, 44) radius 1.6
  circle A11 centre (-22.485, -32.97) radius 0.75
  circle A12 centre (-17.41, -35) radius 0.75
  circle A13 centre (-18.425, -32.97) radius 0.75
  circle A14 centre (-54, -44) radius 1.6
  line L0 (-60, -50) -> (60, -50)
  line L1 (60, -50) -> (60, 50)
  line L2 (60, 50) -> (-60, 50)
  line L3 (-60, 50) -> (-60, -50)
named bodies: "Layer 0", "Layer 1", "Layer 2", "Layer 3", "Layer 4", "Layer 5", "Pin VCC / ESP 16,17,18,21", "Pin CLK / ESP 33", "Pin GND / ESP GND", "Pin MISO / ESP 35"
